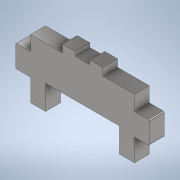
# Autodesk Inventor part: extra_switch_support
Saved by Autodesk Inventor 2020.1 (Build 241239000, 239)
## iProperties
Created: 2019-07-10
Part Number: extra_switch_support
Material: Acier inoxydable
Document SubType Name: Modeling
Designer: Thibault
Density: 8 g/cm^3
Appearance: Semi-poli
Mass: 1.52555 g
Surface Area: 3.13664 cm^2
Volume: 0.190693 cm^3
d18: 2.000 mm
d19: 2.000 mm
d20: 2.000 mm
d21: 2.000 mm
d22: 2.000 mm
d23: 15.00 deg
d24: 15.00 deg
d25: 0.00 deg
d26: 2.000 mm
d27: 2.000 mm
d28: 4.000 mm
d29: 345.00 deg
d30: 330.00 deg
Author: Thibault
Autodesk Inventor part; units mm, degrees
ref_plane "YZ Plane" through (0, 0, 0) normal (1, 0, 0) x (0, 1, 0)
ref_plane "XZ Plane" through (0, 0, 0) normal (0, 1, 0) x (-1, 0, 0)
ref_plane "XY Plane" through (0, 0, 0) normal (0, 0, 1) x (1, 0, 0)
sketch "Unit" plane through (0, 0, 0) normal (0, 0, 1) x (1, 0, 0)
  line L0 (17.4453, 22.2497) -> (21.7153, 22.2497)
  line L1 (21.7153, 22.2497) -> (21.7153, 23.2497)
  line L2 (21.7153, 23.2497) -> (23.4453, 23.2497)
  line L3 (21.7153, 23.2497) -> (21.7153, 24.9797) construction
  line L4 (23.4453, 23.2497) -> (23.4453, 22.6997)
  line L5 (23.4453, 22.6997) -> (25.4453, 22.6997)
  line L6 (25.4453, 22.6997) -> (25.4453, 23.2497)
  line L7 (25.4453, 23.2497) -> (27.1753, 23.2497)
  line L8 (27.1753, 23.2497) -> (27.1753, 22.2497)
  line L9 (27.1753, 22.2497) -> (31.4453, 22.2497)
  line L10 (26.3953, 20.7497) -> (22.4953, 20.7497) construction
  line L11 (22.4953, 20.7497) -> (22.4953, 18.7497) construction
  line L12 (22.4953, 18.7497) -> (26.3953, 18.7497) construction
  line L13 (26.3953, 18.7497) -> (26.3953, 20.7497) construction
  line L14 (26.3953, 20.7497) -> (22.4953, 18.7497) construction
  line L15 (22.4953, 20.7497) -> (26.3953, 18.7497) construction
  point P0 (20.0288, 26.7181)
  point P1 (24.4453, 19.7497)
  dimension "d17" = 2
  dimension "d31" = 110
  dimension "d32" = 0
  dimension "d33" = 2
  dimension "d34" = 20
  dimension "d35" = 20
  dimension "d36" = 1.5
  dimension "d37" = 20.3526
  dimension "d2" = 1
  dimension "d3" = 1.73
  dimension "d4" = 0.55
  dimension "d5" = 2
  dimension "d6" = 1.73
  dimension "d7" = 1
  dimension "d12" = 3.9
  dimension "d13" = 2
  dimension "d14" = 1.5
  dimension "d40" = 14
  measures "d2" distance of L0.end L1.end
  measures "d3" distance of L1.end L2.end
  measures "d4" distance of L2.end L4.end
  measures "d5" distance of L4.end L5.end
  measures "d6" distance of L6.end L7.end
  measures "d7" distance of L7.end L8.end
  measures "d12" distance of L12.end L11.end
  measures "d13" distance of L11.end L10.end
  measures "d14" vertical distance of L0.end L10.end
  measures "d40" distance of L9.end L0.start
sketch "Anchor" plane through (0, 0, 0) normal (0, 0, 1) x (1, 0, 0)
  line L0 (2, 0) -> (2, 1.875)
  line L1 (2, 0) -> (3, 0) construction
  line L2 (2.125, 2) -> (4.875, 2)
  line L3 (5, 1.875) -> (5, 0)
  line L4 (5, 2) -> (7, 2) construction
  line L5 (0, 0) -> (2, 0)
  line L6 (5, 0) -> (7, 0)
  arc A0 (2.125, 2) -> (2, 1.875) centre (2.125, 1.875) ccw
  arc A1 (5, 1.875) -> (4.875, 2) centre (4.875, 1.875) ccw
  point P0 (9.1321, -0.6227)
  point P1 (2, 2)
  dimension "d69" = 15
  dimension "d45" = 2
  dimension "d46" = 2
  dimension "d47" = 3
  dimension "d48" = 2
  dimension "d60" = 2
  dimension "d67" = 0.125
  measures "d45" distance of point (0, 0) L0.start
  measures "d46" distance of L0.start point (2, 2)
  measures "d47" distance of point (2, 2) L4.start
  measures "d48" distance of L3.end L4.start
  measures "d60" distance of L3.end point (7, 0)
  measures "d67" radius of A0
sketch "Esquisse2" plane through (0, 0, 0) normal (0, 0, 1) x (1, 0, 0)
  line L0 (-10.7801, -14.9425) -> (-8.7801, -14.9425)
  line L1 (-10.7801, -13.9425) -> (-10.7801, -14.9425)
  line L2 (3.2199, -13.9425) -> (3.2199, -14.9425)
  line L3 (-8.7801, -14.9425) -> (-8.7801, -11.6425)
  line L4 (1.2199, -11.6425) -> (1.2199, -14.9425)
  line L5 (1.2199, -14.9425) -> (3.2199, -14.9425)
  line L6 (-8.7801, -11.6425) -> (1.2199, -11.6425)
  line L7 (-10.7801, -11.9425) -> (-12.6551, -11.9425)
  line L8 (-10.7801, -11.9425) -> (-10.7801, -10.9425) construction
  line L9 (-12.7801, -11.8175) -> (-12.7801, -9.0675)
  line L10 (-12.6551, -8.9425) -> (-10.7801, -8.9425)
  line L11 (-12.7801, -8.9425) -> (-12.7801, -6.9425) construction
  line L12 (-10.7801, -13.9425) -> (-10.7801, -11.9425)
  line L13 (-10.7801, -8.9425) -> (-10.7801, -6.9425)
  arc A0 (-12.7801, -11.8175) -> (-12.6551, -11.9425) centre (-12.6551, -11.8175) ccw
  arc A1 (-12.6551, -8.9425) -> (-12.7801, -9.0675) centre (-12.6551, -9.0675) ccw
  line L14 (3.2199, -8.9425) -> (5.0949, -8.9425)
  line L15 (3.2199, -8.9425) -> (3.2199, -9.9425) construction
  line L16 (5.2199, -9.0675) -> (5.2199, -11.8175)
  line L17 (5.0949, -11.9425) -> (3.2199, -11.9425)
  line L18 (5.2199, -11.9425) -> (5.2199, -13.9425) construction
  line L19 (3.2199, -6.9425) -> (3.2199, -8.9425)
  line L20 (3.2199, -11.9425) -> (3.2199, -13.9425)
  arc A2 (5.2199, -9.0675) -> (5.0949, -8.9425) centre (5.0949, -9.0675) ccw
  arc A3 (5.0949, -11.9425) -> (5.2199, -11.8175) centre (5.0949, -11.8175) ccw
  line L21 (-10.7801, -6.9425) -> (-6.5101, -6.9425)
  line L22 (-6.5101, -6.9425) -> (-6.5101, -5.9425)
  line L23 (-6.5101, -5.9425) -> (-4.7801, -5.9425)
  line L24 (-6.5101, -5.9425) -> (-6.5101, -4.2125) construction
  line L25 (-4.7801, -5.9425) -> (-4.7801, -6.4925)
  line L26 (-4.7801, -6.4925) -> (-2.7801, -6.4925)
  line L27 (-2.7801, -6.4925) -> (-2.7801, -5.9425)
  line L28 (-2.7801, -5.9425) -> (-1.0501, -5.9425)
  line L29 (-1.0501, -5.9425) -> (-1.0501, -6.9425)
  line L30 (-1.0501, -6.9425) -> (3.2199, -6.9425)
  line L31 (-1.8301, -8.4425) -> (-5.7301, -8.4425) construction
  line L32 (-5.7301, -8.4425) -> (-5.7301, -10.4425) construction
  line L33 (-5.7301, -10.4425) -> (-1.8301, -10.4425) construction
  line L34 (-1.8301, -10.4425) -> (-1.8301, -8.4425) construction
  line L35 (-1.8301, -8.4425) -> (-5.7301, -10.4425) construction
  line L36 (-5.7301, -8.4425) -> (-1.8301, -10.4425) construction
  point P0 (0, 0)
  point P1 (3.2199, -6.9425)
  point P2 (-10.7801, -6.9425)
  point P3 (-10.7803, -12.8535)
  point P4 (3.2197, -12.8535)
  dimension "d101" = 14
  dimension "d97" = 4.7
  dimension "d98" = 8
  dimension "d99" = 2
  dimension "d100" = 10
  constraints: 14 end point, 3 vertical, 2 collinear, 2 horizontal, 2 other
  measures "d99" distance of L0.start L0.end
  measures "d100" distance of L3.end L4.start
extrude "Extrusion1" add sketch "Esquisse2" along normal blind 2
equation "\"d35\" = d34"
equation "\"d6\" = d3"
equation "\"d7\" = d2"
equation "\"d13\" = sheet_thickness"
equation "\"d45\" = safe_distance"
equation "\"d46\" = sheet_thickness"
equation "\"d47\" = 1.5 * sheet_thickness"
equation "\"d48\" = sheet_thickness"
equation "\"d99\" = safe_distance"
equation "\"d71\" = sheet_thickness"
equation "\"d60\" = safe_distance"
equation "\"sheet_thickness\" = 2"
equation "\"safe_distance\" = 2"
